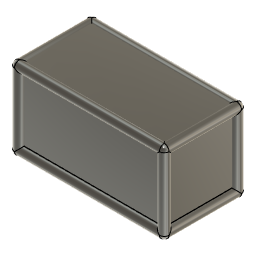
2022_10_03_Arena Drone Soccer Ball (not official) v1 (Autodesk Fusion 360 design; units mm, degrees)
Autodesk Fusion 360 part; units mm, degrees
sketch "Sketch1" plane through (0, 0, 0) normal (0, 0, 1) x (1, 0, 0)
  line L0 (300, 150) -> (-300, 150)
  line L1 (-300, 150) -> (-300, -150)
  line L2 (-300, -150) -> (300, -150)
  line L3 (300, -150) -> (300, 150)
  line L4 (300, 150) -> (-300, -150) construction
  line L5 (-300, 150) -> (300, -150) construction
  circle A0 centre (-300, 150) radius 20
  circle A1 centre (300, 150) radius 20
  circle A2 centre (300, -150) radius 20
  circle A3 centre (-300, -150) radius 20
  line L6 (-300, 150) -> (-300, 170)
  dimension "d1" = 600
  dimension "d2" = 300
  dimension "d3" = 40
  constraint horizontal L0
  constraint perpendicular L0 L1
  constraint parallel L0 L2
  constraint parallel L1 L3
  constraint coincident L4 origin
  constraint coincident L5 origin
  constraint coincident L0.end L1.start
  constraint coincident L0.start L3.end
  constraint coincident L2.end L3.start
  constraint coincident L1.end L2.start
  constraint equal A0 A1
  constraint equal A0 A2
  constraint equal A0 A3
  constraint coincident A0 L6.end
  constraint parallel L1 L6
  measures "d1" distance of L1.end L2.end
  measures "d2" distance of L0.end L1.end
  measures "d3" diameter of A0
extrude "Extrude1" add sketch "Sketch1" along normal blind 300 contours L0 L1 A0 | L0 A0 L6 | L1 A0 L6 | L0 L3 A1 | L0 L3 A1 | L1 L2 A3 | L1 L2 A3 | L2 L3 A2 | L2 L3 A2 makes body 1 at (-280.0994, -148.0086, 200) makes body 2 at (319.9006, -148.0086, 200) makes body 3 at (-280.0994, 151.9914, 200) makes body 4 at (319.9006, 151.9914, 200)
extrude "Extrude2" add sketch "Sketch1" along normal blind 600 separate body contours L0 L1 A0 | L0 A0 L6 | L1 A0 L6 | L1 L2 A3 | L1 L2 A3 makes body 5 at (-280.0994, 151.9914, 400) makes body 6 at (-280.0994, -148.0086, 400)
extrude "Extrude3" add sketch "Sketch1" along normal blind 300 separate body contours L0 L1 A0 | L0 A0 L6 | L1 A0 L6 | L0 L3 A1 | L0 L3 A1 makes body 7 at (319.9006, 151.9914, 200) makes body 8 at (-280.0994, 151.9914, 200)
move_body "Move3" bodies 5 6 to x (0, 0, -1) y (0, 1, 0) z (1, 0, 0) at (-300, 0, -300)
move_body "Move4" bodies 7 3 to x (1, 0, 0) y (0, 0, 1) z (0, -1, 0) at (0, 150, -150)
copy_body "CopyPasteBodies2" bodies 3 5 7 6 makes body 9 makes body 10 makes body 11 makes body 12
move_body "Move5" bodies 9 10 11 12 to x (1, 0, 0) y (0, 1, 0) z (0, 0, 1) at (0, 0, 300)
revolve "Revolve1" add sketch "Sketch1" angle 360 about axis through (-300, 150, 0) along (0, 1, 0) separate body contours L1 A0 L6 makes body 13
copy_body "CopyPasteBodies3" bodies 13 makes body 14
move_body "Move6" bodies 14 to x (1, 0, 0) y (0, 1, 0) z (0, 0, 1) at (0, 0, 300)
move_body "Move7" bodies 14 13 to x (1, 0, 0) y (0, 1, 0) z (0, 0, 1) at (0, -300, 0)
copy_body "CopyPasteBodies4" bodies 13 14 makes body 15 makes body 16
move_body "Move8" bodies 15 16 to x (1, 0, 0) y (0, 1, 0) z (0, 0, 1) at (0, 300, 0)
copy_body "CopyPasteBodies5" bodies 16 13 14 15 makes body 17 makes body 18 makes body 19 makes body 20
move_body "Move9" bodies 17 18 19 20 to x (1, 0, 0) y (0, 1, 0) z (0, 0, 1) at (600, 0, 0)
combine "Combine1" operation add target body 1 tool bodies 4 5 19 13 18 20 10 7 9 16 8 11 12 14 17 15 3 2 6
move_body "Move10" bodies 1 to x (1, 0, 0) y (0, 1, 0) z (0, 0, 1) at (0, 0, -20)
extrude "Extrude4" add sketch "Sketch1" against normal blind 1 separate body contours L0 L1 L2 L3 A0 A1 A2 A3 makes body 21
sketch "Sketch2" plane through (0, 0, 0) normal (1, 0, 0) x (0, 1, 0)
  line L0 (-150, 275) -> (150, 275)
  line L1 (150, 275) -> (150, -25)
  line L2 (150, -25) -> (-150, -25)
  line L3 (-150, -25) -> (-150, 275)
  line L4 (-150, 275) -> (150, -25) construction
  line L5 (150, 275) -> (-150, -25) construction
  point P0 (0, 125)
  constraint horizontal L0
  constraint perpendicular L0 L1
  constraint parallel L0 L2
  constraint parallel L1 L3
  constraint coincident L4 P0
  constraint coincident L5 P0
sketch "Sketch3" plane through (0, 0, 0) normal (0, 1, 0) x (1, 0, 0)
  line L0 (-300.7275, -286.7995) -> (300.7275, -286.7995)
  line L1 (300.7275, -286.7995) -> (300.7275, 36.7995)
  line L2 (300.7275, 36.7995) -> (-300.7275, 36.7995)
  line L3 (-300.7275, 36.7995) -> (-300.7275, -286.7995)
  line L4 (-300.7275, -286.7995) -> (300.7275, 36.7995) construction
  line L5 (300.7275, -286.7995) -> (-300.7275, 36.7995) construction
  point P0 (0, -125)
  constraint horizontal L0
  constraint perpendicular L0 L1
  constraint parallel L0 L2
  constraint parallel L1 L3
  constraint coincident L4 P0
  constraint coincident L5 P0
extrude "Extrude5" add sketch "Sketch3" along normal blind 1 separate body makes body 22
extrude "Extrude6" add sketch "Sketch2" along normal blind 1 separate body makes body 23
move_body "Move11" bodies 23 to x (1, 0, 0) y (0, 1, 0) z (0, 0, 1) at (-300, 0, 0)
move_body "Move12" bodies 22 to x (1, 0, 0) y (0, 1, 0) z (0, 0, 1) at (0, 150, 0)
copy_body "CopyPasteBodies6" bodies 23 makes body 24
move_body "Move13" bodies 24 to x (1, 0, 0) y (0, 1, 0) z (0, 0, 1) at (600, 0, 0)
move_body "Move14" bodies 22 to x (1, 0, 0) y (0, 1, 0) z (0, 0, 1) at (0, -300, 0)
copy_body "CopyPasteBodies7" bodies 22 makes body 25
move_body "Move15" bodies 25 to x (1, 0, 0) y (0, 1, 0) z (0, 0, 1) at (0, 300, 0)
sketch "Sketch4" plane through (0, 0, 0) normal (0, 0, 1) x (1, 0, 0)
  line L0 (300, 150) -> (-300, 150)
  line L1 (-300, 150) -> (-300, -150)
  line L2 (-300, -150) -> (300, -150)
  line L3 (300, -150) -> (300, 150)
  line L4 (300, 150) -> (-300, -150) construction
  line L5 (-300, 150) -> (300, -150) construction
  constraint horizontal L0
  constraint perpendicular L0 L1
  constraint parallel L0 L2
  constraint parallel L1 L3
  constraint coincident L4 origin
  constraint coincident L5 origin
extrude "Extrude7" add sketch "Sketch4" along normal blind 1 separate body makes body 26
move_body "Move16" bodies 26 to x (1, 0, 0) y (0, 1, 0) z (0, 0, 1) at (0, 0, 295)
named bodies: "Borders", "Down", "Right", "Front", "Back", "Left", "Top"
